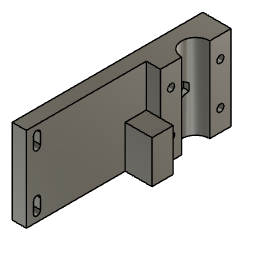
Pump Clamp v1.0 (Autodesk Fusion 360 design; units mm, degrees)
Autodesk Fusion 360 part; units mm, degrees
sketch "Sketch1" plane through (0, 0, 0) normal (0, 0, 1) x (1, 0, 0)
  circle A0 centre (0, 0) radius 10
  line L0 (0, 0) -> (0, 10) construction
  line L1 (0, 10) -> (0, 25)
  line L2 (0, 25) -> (-20, 25)
  line L3 (-20, 25) -> (-20, -25)
  line L4 (-20, -25) -> (0, -25)
  line L5 (0, -25) -> (0, -10)
  line L6 (-20, -25) -> (-20, -110)
  line L7 (-20, -110) -> (-10, -110)
  line L8 (-10, -110) -> (-10, -25)
  line L9 (-10, -25) -> (9, -25)
  line L10 (9, -25) -> (9, -40)
  line L11 (9, -40) -> (-10, -40)
  line L12 (-10, -40) -> (-10, -25)
  dimension "d1" = 20
  dimension "d2" = 15
  dimension "d3" = 20
  dimension "d4" = 50
  dimension "d5" = 85
  dimension "d6" = 10
  dimension "d7" = 19
  constraint coincident A0.centre L0.start
  constraint coincident A0 L0.end
  constraint vertical L0
  constraint parallel L0 L1
  constraint perpendicular L1 L2
  constraint perpendicular L2 L3
  constraint perpendicular L3 L4
  constraint coincident A0 L5.end
  constraint perpendicular L4 L5
  constraint perpendicular L4 L6
  constraint perpendicular L6 L7
  constraint midpoint L4 L8.end
  constraint perpendicular L4 L8
  constraint horizontal L9
  constraint vertical L10
  constraint horizontal L11
  constraint vertical L12
  measures "d1" diameter of A0
  measures "d2" distance of L0.end L1.end
  measures "d3" distance of L1.end L2.end
  measures "d4" distance of L2.end L3.end
  measures "d5" distance of L3.end L6.end
  measures "d6" distance of L6.end L7.end
  measures "d7" distance of L8.end L9.end
extrude "Extrude1" add sketch "Sketch1" along normal blind 60 contours A0 L1 L2 L3 L4 L5 L9
extrude "Extrude2" add sketch "Sketch1" along normal blind 30 contours L4 L8 L9 L10 L11 L12
extrude "Extrude3" add sketch "Sketch1" along normal blind 60 contours L4 L6 L7 L8 L12
sketch "Sketch2" plane through (-20, 0, 0) normal (-1, 0, 0) x (0, -1, 0)
  line L0 (-25, 0) -> (110, 0)
  line L1 (110, 0) -> (110, 60)
  line L2 (110, 60) -> (-25, 60)
  line L3 (-25, 60) -> (-25, 0)
  line L4 (-25, 60) -> (-17.5, 60) construction
  line L5 (-17.5, 60) -> (27.5, 60) construction
  line L6 (-17.5, 60) -> (-17.5, 45) construction
  circle A0 centre (-17.5, 15) radius 2.5
  line L7 (110, 30) -> (102.5, 30) construction
  line L8 (102.5, 30) -> (102.5, 46.25) construction
  circle A1 centre (102.5, 46.25) radius 2.5
  circle A2 centre (102.5, 53.75) radius 2.5
  line L9 (102.5, 53.75) -> (100, 53.75) construction
  line L10 (102.5, 46.25) -> (100, 46.25) construction
  line L11 (100, 53.75) -> (100, 46.25)
  line L12 (105, 53.75) -> (105, 46.25)
  circle A3 centre (102.5, 6.25) radius 2.5
  line L13 (105, 6.25) -> (105, 13.75)
  circle A4 centre (102.5, 13.75) radius 2.5
  line L14 (100, 6.25) -> (100, 13.75)
  circle A5 centre (17.5, 15) radius 2.5
  circle A6 centre (-17.5, 45) radius 2.5
  circle A7 centre (17.5, 45) radius 2.5
  line L15 (-17.5, 45) -> (17.5, 45) construction
  line L16 (-17.5, 15) -> (17.5, 15) construction
  line L17 (0, 15) -> (0, 45) construction
  circle A8 centre (0, 30) radius 2.5
  dimension "d14" = 7.5
  dimension "d15" = 45
  dimension "d16" = 15
  dimension "d23" = 7.5
  dimension "d24" = 16.25
  dimension "d25" = 5
  dimension "d28" = 0
  dimension "d29" = 7.5
  dimension "d34" = 35
  dimension "d35" = 30
  dimension "d36" = 5
  constraint coincident L2.end L3.start
  constraint perpendicular L3 L4
  constraint parallel L4 L5
  constraint perpendicular L4 L6
  constraint midpoint L1 L7.start
  constraint perpendicular L1 L7
  constraint perpendicular L7 L8
  constraint coincident L8.end A1.centre
  constraint coincident A2.centre L9.start
  constraint coincident A2 L9.end
  constraint horizontal L9
  constraint coincident A1 L10.end
  constraint perpendicular L8 L10
  constraint coincident A2 L12.start
  constraint coincident A1 L12.end
  constraint tangent A1 L12
  constraint parallel L11 L12
  constraint symmetric L7 A1 A4
  constraint symmetric L7 A2 A3
  constraint symmetric L7 L9.end L14.start
  constraint symmetric L7 L10.end L14.end
  constraint symmetric L7 L12.start L13.start
  constraint symmetric L7 L12.end L13.end
  constraint coincident A7.centre L15.end
  constraint perpendicular L3 L15
  constraint coincident A0.centre L16.start
  constraint coincident A5.centre L16.end
  constraint midpoint L16 L17.start
  constraint midpoint L15 L17.end
  constraint perpendicular L15 L17
  constraint midpoint L17 A8.centre
  measures "d14" distance of L2.end L4.end
  measures "d15" distance of L4.end L5.end
  measures "d16" distance of L4.end L6.end
  measures "d23" distance of L7.start L7.end
  measures "d24" distance of L7.end L8.end
  measures "d25" diameter of A1
  measures "d36" diameter of A8
extrude "Extrude4" cut sketch "Sketch2" against normal blind 20 contours A0 | A1 | A1 A2 L11 L12 | A2 | A3 | A3 L13 A4 L14 | A4 | A5 | A6 | A7 | A8
sketch "Sketch3" plane through (-20, 0, 0) normal (-1, 0, 0) x (0, -1, 0)
  circle A0 centre (17.5, 45) radius 2.5
  circle A1 centre (-17.5, 45) radius 2.5
  circle A2 centre (17.5, 15) radius 2.5
  arc A3 (105, 13.75) -> (100, 13.75) centre (102.5, 13.75) ccw
  line L0 (105, 13.75) -> (105, 6.25)
  arc A4 (100, 6.25) -> (105, 6.25) centre (102.5, 6.25) ccw
  line L1 (100, 6.25) -> (100, 13.75)
  circle A5 centre (-17.5, 15) radius 2.5
  circle A6 centre (0, 30) radius 2.5
  arc A7 (100, 46.25) -> (105, 46.25) centre (102.5, 46.25) ccw
  line L2 (100, 46.25) -> (100, 53.75)
  arc A8 (105, 53.75) -> (100, 53.75) centre (102.5, 53.75) ccw
  line L3 (105, 53.75) -> (105, 46.25)
  line L4 (-25, 0) -> (110, 0)
  line L5 (110, 0) -> (110, 60)
  line L6 (110, 60) -> (-25, 60)
  line L7 (-25, 60) -> (-25, 0)
  circle A9 centre (-17.5, 45) radius 5
  circle A10 centre (17.5, 45) radius 5
  circle A11 centre (-17.5, 15) radius 5
  circle A12 centre (17.5, 15) radius 5
  line L8 (0, 30) -> (0, 35) construction
  line L9 (0, 35) -> (-4.3301, 32.5)
  line L10 (-4.3301, 32.5) -> (-4.3301, 27.5)
  line L11 (-4.3301, 27.5) -> (0, 25)
  line L12 (0, 25) -> (4.3301, 27.5)
  line L13 (4.3301, 27.5) -> (4.3301, 32.5)
  line L14 (4.3301, 32.5) -> (0, 35)
  point P0 (0, 30)
  dimension "d37" = 10
  dimension "d40" = 35
  dimension "d41" = -30
  dimension "d42" = 5
  constraint concentric A1 A9
  constraint coincident P0 A6.centre
  constraint vertical L8
  constraint coincident L8.end L9.start
  measures "d37" diameter of A9
  measures "d42" distance of P0 L8.end
extrude "Extrude5" cut sketch "Sketch3" against normal blind 5 contours A9 | A10 | A11 | A12
extrude "Extrude6" cut sketch "Sketch3" against normal blind 6 from surface at -7 contours L9 L10 L11 L12 L13 L14
